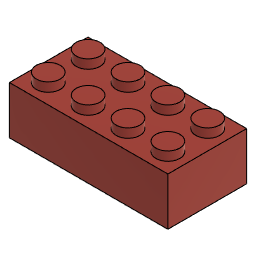
Red Brick v1 (Autodesk Fusion 360 design; units mm, degrees)
Autodesk Fusion 360 part; units mm, degrees
sketch "side" plane through (0, 0, 0) normal (1, 0, 0) x (0, 1, 0)
  line L0 (0, 0) -> (15.8, 0)
  line L1 (15.8, 0) -> (15.8, 9.6)
  line L2 (15.8, 9.6) -> (0, 9.6)
  line L3 (0, 9.6) -> (0, 0)
  dimension "d1" = 15.8
  dimension "d2" = 9.6
  constraint horizontal L0
  constraint vertical L1
  constraint horizontal L2
  constraint vertical L3
  constraint coincident L0.start L3.end
  measures "d1" distance of L0.start L0.end
  measures "d2" distance of L0 L2
sketch "top" plane through (0, 0, 0) normal (0, 0, 1) x (1, 0, 0)
  line L0 (0, 0) -> (-31.8, 0)
  line L1 (-31.8, 0) -> (-31.8, 15.8)
  line L2 (-31.8, 15.8) -> (0, 15.8)
  line L3 (0, 15.8) -> (0, 0)
  circle A0 centre (-3.9, 11.9) radius 2.4
  line L4 (0, 15.8) -> (0, 0)
  circle A1 centre (-11.9, 11.9) radius 2.4
  circle A2 centre (-19.9, 11.9) radius 2.4
  circle A3 centre (-27.9, 11.9) radius 2.4
  circle A4 centre (-3.9, 3.9) radius 2.4
  circle A5 centre (-11.9, 3.9) radius 2.4
  circle A6 centre (-19.9, 3.9) radius 2.4
  circle A7 centre (-27.9, 3.9) radius 2.4
  circle A8 centre (-7.9, 7.9) radius 3.255
  circle A9 centre (-7.9, 7.9) radius 2.4
  circle A10 centre (-3.9, 11.9) radius 1.3
  circle A11 centre (-3.9, 3.9) radius 1.3
  circle A12 centre (-11.9, 11.9) radius 1.3
  circle A13 centre (-11.9, 3.9) radius 1.3
  circle A14 centre (-19.9, 11.9) radius 1.3
  circle A15 centre (-19.9, 3.9) radius 1.3
  circle A16 centre (-27.9, 11.9) radius 1.3
  circle A17 centre (-27.9, 3.9) radius 1.3
  circle A18 centre (-15.9, 7.9) radius 3.255
  circle A19 centre (-23.9, 7.9) radius 3.255
  circle A20 centre (-15.9, 7.9) radius 2.4
  circle A21 centre (-23.9, 7.9) radius 2.4
  line L5 (-30.6, 14.6) -> (-1.2, 14.6)
  line L6 (-1.2, 14.6) -> (-1.2, 1.2)
  line L7 (-1.2, 1.2) -> (-30.6, 1.2)
  line L8 (-30.6, 1.2) -> (-30.6, 14.6)
  line L9 (-15.9, 7.9) -> (-15.9, 14.6) construction
  line L10 (-15.9, 7.9) -> (-15.9, 1.2) construction
  line L11 (-16.3, 11.1303) -> (-16.3, 14.6)
  line L12 (-15.5, 11.1303) -> (-15.5, 14.6)
  line L13 (-15.5, 4.6697) -> (-15.5, 1.2)
  line L14 (-16.3, 4.6697) -> (-16.3, 1.2)
  line L15 (-28.2, 14.6) -> (-27.6, 14.6)
  line L16 (-27.6, 14.6) -> (-27.6, 14.4)
  line L17 (-27.6, 14.4) -> (-28.2, 14.4)
  line L18 (-28.2, 14.4) -> (-28.2, 14.6)
  line L19 (-20.2, 14.6) -> (-19.6, 14.6)
  line L20 (-19.6, 14.6) -> (-19.6, 14.4)
  line L21 (-19.6, 14.4) -> (-20.2, 14.4)
  line L22 (-20.2, 14.4) -> (-20.2, 14.6)
  line L23 (-12.2, 14.6) -> (-11.6, 14.6)
  line L24 (-11.6, 14.6) -> (-11.6, 14.4)
  line L25 (-11.6, 14.4) -> (-12.2, 14.4)
  line L26 (-12.2, 14.4) -> (-12.2, 14.6)
  line L27 (-4.2, 14.4) -> (-3.6, 14.4)
  line L28 (-3.6, 14.4) -> (-3.6, 14.6)
  line L29 (-3.6, 14.6) -> (-4.2, 14.6)
  line L30 (-4.2, 14.6) -> (-4.2, 14.4)
  line L31 (-1.4, 12.2) -> (-1.2, 12.2)
  line L32 (-1.2, 12.2) -> (-1.2, 11.6)
  line L33 (-1.2, 11.6) -> (-1.4, 11.6)
  line L34 (-1.4, 11.6) -> (-1.4, 12.2)
  line L35 (-1.4, 4.2) -> (-1.2, 4.2)
  line L36 (-1.2, 4.2) -> (-1.2, 3.6)
  line L37 (-1.2, 3.6) -> (-1.4, 3.6)
  line L38 (-1.4, 3.6) -> (-1.4, 4.2)
  line L39 (-4.2, 1.4) -> (-3.6, 1.4)
  line L40 (-3.6, 1.4) -> (-3.6, 1.2)
  line L41 (-3.6, 1.2) -> (-4.2, 1.2)
  line L42 (-4.2, 1.2) -> (-4.2, 1.4)
  line L43 (-11.6, 1.4) -> (-12.2, 1.4)
  line L44 (-12.2, 1.4) -> (-12.2, 1.2)
  line L45 (-12.2, 1.2) -> (-11.6, 1.2)
  line L46 (-11.6, 1.2) -> (-11.6, 1.4)
  line L47 (-19.6, 1.4) -> (-20.2, 1.4)
  line L48 (-20.2, 1.4) -> (-20.2, 1.2)
  line L49 (-20.2, 1.2) -> (-19.6, 1.2)
  line L50 (-19.6, 1.2) -> (-19.6, 1.4)
  line L51 (-27.6, 1.4) -> (-28.2, 1.4)
  line L52 (-28.2, 1.4) -> (-28.2, 1.2)
  line L53 (-28.2, 1.2) -> (-27.6, 1.2)
  line L54 (-27.6, 1.2) -> (-27.6, 1.4)
  line L55 (-30.4, 4.2) -> (-30.6, 4.2)
  line L56 (-30.6, 4.2) -> (-30.6, 3.6)
  line L57 (-30.6, 3.6) -> (-30.4, 3.6)
  line L58 (-30.4, 3.6) -> (-30.4, 4.2)
  line L59 (-30.4, 12.2) -> (-30.6, 12.2)
  line L60 (-30.6, 12.2) -> (-30.6, 11.6)
  line L61 (-30.6, 11.6) -> (-30.4, 11.6)
  line L62 (-30.4, 11.6) -> (-30.4, 12.2)
  dimension "d3" = 31.8
  dimension "d4" = 15.8
  dimension "d5" = 4.8
  dimension "d6" = 3.9
  dimension "d7" = 3.9
  dimension "d8" = 4.8
  dimension "d9" = 4.8
  dimension "d10" = 4.8
  dimension "d11" = 4.8
  dimension "d12" = 4.8
  dimension "d13" = 4.8
  dimension "d14" = 4.8
  dimension "d15" = 3.9
  dimension "d16" = 3.9
  dimension "d17" = 3.9
  dimension "d18" = 8
  dimension "d19" = 8
  dimension "d20" = 8
  dimension "d21" = 8
  dimension "d22" = 8
  dimension "d23" = 8
  dimension "d24" = 3.9
  dimension "d25" = 8
  dimension "d26" = 8
  dimension "d27" = 8
  dimension "d28" = 8
  dimension "d29" = 6.51
  dimension "d30" = 7.9
  dimension "d31" = 7.9
  dimension "d32" = 4.8
  dimension "d33" = 2.6
  dimension "d34" = 2.6
  dimension "d35" = 2.6
  dimension "d36" = 2.6
  dimension "d37" = 2.6
  dimension "d38" = 2.6
  dimension "d39" = 2.6
  dimension "d40" = 2.6
  dimension "d41" = 6.51
  dimension "d42" = 6.51
  dimension "d43" = 8
  dimension "d44" = 7.9
  dimension "d45" = 8
  dimension "d46" = 7.9
  dimension "d47" = 4.8
  dimension "d48" = 4.8
  dimension "d49" = 1.2
  dimension "d50" = 1.2
  dimension "d51" = 1.2
  dimension "d52" = 1.2
  dimension "d53" = 0.8
  dimension "d54" = 0.4
  dimension "d55" = 0.4
  dimension "d56" = 0.8
  dimension "d57" = 0.6
  dimension "d58" = 0.2
  dimension "d60" = 0.6
  dimension "d61" = 0.3
  dimension "d62" = 0.6
  dimension "d63" = 0.3
  dimension "d64" = 0.6
  dimension "d65" = 0.3
  dimension "d66" = 0.6
  dimension "d67" = 0.3
  dimension "d68" = 0.6
  dimension "d69" = 0.6
  dimension "d70" = 0.6
  dimension "d71" = 0.6
  dimension "d72" = 0.6
  dimension "d73" = 0.6
  dimension "d74" = 0.3
  dimension "d75" = 0.6
  constraint horizontal L0
  constraint vertical L1
  constraint horizontal L2
  constraint vertical L3
  constraint coincident L0.start L3.end
  constraint concentric A8 A9
  constraint concentric A0 A10
  constraint concentric A4 A11
  constraint concentric A1 A12
  constraint concentric A5 A13
  constraint concentric A2 A14
  constraint concentric A6 A15
  constraint concentric A3 A16
  constraint concentric A7 A17
  constraint concentric A18 A20
  constraint concentric A19 A21
  constraint horizontal L5
  constraint vertical L6
  constraint horizontal L7
  constraint vertical L8
  constraint coincident A18.centre A20.centre
  constraint midpoint L5 L9.end
  constraint midpoint L7 L10.end
  constraint coincident A18 L11.start
  constraint coincident L5 L11.end
  constraint perpendicular L5 L11
  constraint coincident A18 L12.start
  constraint coincident L5 L12.end
  constraint perpendicular L5 L12
  constraint coincident A18 L13.start
  constraint coincident L7 L13.end
  constraint perpendicular L7 L13
  constraint coincident A18 L14.start
  constraint coincident L7 L14.end
  constraint perpendicular L7 L14
  constraint horizontal L15
  constraint vertical L16
  constraint horizontal L17
  constraint vertical L18
  constraint coincident L5 L15.start
  constraint horizontal L19
  constraint vertical L20
  constraint horizontal L21
  constraint vertical L22
  constraint coincident L5 L19.start
  constraint horizontal L23
  constraint vertical L24
  constraint horizontal L25
  constraint vertical L26
  constraint coincident L5 L23.start
  constraint horizontal L27
  constraint vertical L28
  constraint horizontal L29
  constraint vertical L30
  constraint horizontal L31
  constraint vertical L32
  constraint horizontal L33
  constraint vertical L34
  constraint horizontal L35
  constraint vertical L36
  constraint horizontal L37
  constraint vertical L38
  constraint horizontal L39
  constraint vertical L40
  constraint horizontal L41
  constraint vertical L42
  constraint horizontal L43
  constraint vertical L44
  constraint horizontal L45
  constraint vertical L46
  constraint horizontal L47
  constraint vertical L48
  constraint horizontal L49
  constraint vertical L50
  constraint coincident L7 L48.end
  constraint horizontal L51
  constraint vertical L52
  constraint horizontal L53
  constraint vertical L54
  constraint horizontal L55
  constraint vertical L56
  constraint horizontal L57
  constraint vertical L58
  constraint horizontal L59
  constraint vertical L60
  constraint horizontal L61
  constraint vertical L62
  measures "d3" distance of L0.start L0.end
  measures "d4" distance of L0.start L2.end
  measures "d5" diameter of A0
  measures "d6" distance of L2 A0.centre
  measures "d7" distance of A0.centre L4
  measures "d8" diameter of A1
  measures "d9" diameter of A2
  measures "d10" diameter of A3
  measures "d11" diameter of A4
  measures "d12" diameter of A5
  measures "d13" diameter of A6
  measures "d14" diameter of A7
  measures "d15" distance of L2 A1.centre
  measures "d16" distance of L2 A2.centre
  measures "d17" distance of L2 A3.centre
  measures "d18" horizontal distance of A4.centre A5.centre
  measures "d19" horizontal distance of A1.centre A4.centre
  measures "d20" distance of A1.centre A2.centre
  measures "d21" distance of A2.centre A3.centre
  measures "d22" horizontal distance of A6.centre A7.centre
  measures "d23" horizontal distance of A5.centre A6.centre
  measures "d24" distance of L4 A4.centre
  measures "d25" distance of A3.centre A7.centre
  measures "d26" distance of A0.centre A4.centre
  measures "d27" distance of A1.centre A5.centre
  measures "d28" distance of A2.centre A6.centre
  measures "d29" diameter of A8
  measures "d30" distance of L2 A8.centre
  measures "d31" distance of L4 A8.centre
  measures "d32" diameter of A9
  measures "d33" diameter of A10
  measures "d34" diameter of A11
  measures "d35" diameter of A12
  measures "d36" diameter of A13
  measures "d37" diameter of A14
  measures "d38" diameter of A15
  measures "d39" diameter of A16
  measures "d40" diameter of A17
  measures "d41" diameter of A18
  measures "d42" diameter of A19
  measures "d43" horizontal distance of A8.centre A18.centre
  measures "d44" distance of L2 A18.centre
  measures "d45" horizontal distance of A18.centre A19.centre
  measures "d46" distance of L2 A19.centre
  measures "d47" diameter of A20
  measures "d48" diameter of A21
  measures "d49" distance of L1 L8
  measures "d50" distance of L4 L6
  measures "d51" distance of L2 L5
  measures "d52" distance of L0 L7
  measures "d53" distance of L11 L12
  measures "d54" distance of L9 L12
  measures "d55" distance of L10 L13
  measures "d56" distance of L13 L14
  measures "d57" distance of L15.start L15.end
  measures "d58" distance of L15 L17
  measures "d60" distance of L19.start L19.end
  measures "d61" distance of A2.centre L20
  measures "d62" distance of L23.start L23.end
  measures "d63" distance of A1.centre L24
  measures "d64" distance of L27.start L27.end
  measures "d65" distance of A0.centre L28
  measures "d66" distance of L31.start L33.end
  measures "d67" distance of A0.centre L31
  measures "d68" distance of L35.start L37.end
  measures "d69" distance of L39.start L39.end
  measures "d70" distance of L43.start L43.end
  measures "d71" distance of L47.start L47.end
  measures "d72" distance of L51.start L51.end
  measures "d73" distance of L55.start L57.end
  measures "d74" distance of A7.centre L55
  measures "d75" distance of L59.start L61.end
extrude "Extrude1" add sketch "top" along normal blind 9.6 contours L0 L1 L2 L3 L4 | L5 L23 L24 L25 L26 | L5 L19 L20 L21 L22 | L7 L43 L44 L45 L46 | L5 L27 L28 L29 L30 | L7 L47 L48 L49 L50 | L5 L15 L16 L17 L18 | L7 L39 L40 L41 L42 | L7 L51 L52 L53 L54 | L6 L31 L32 L33 L34 | L8 L59 L60 L61 L62 | L6 L35 L36 L37 L38 | L8 L55 L56 L57 L58 makes body 1
extrude "Extrude2" add sketch "top" along normal blind 9.6 and the other way blind -8.6 contours A0 | A4 | A1 A5 A8 A18 L5 L6 L7 L12 L13 L24 L25 L26 L27 L28 L30 L31 L33 L34 L35 L37 L38 L39 L40 L42 L43 L44 L46 | A8 | A1 A5 A8 A18 | A1 | A18 | A5 | A18 L5 L11 L12 | A7 | A3 | A2 A6 A18 A19 L5 L7 L8 L11 L14 L16 L17 L18 L20 L21 L22 L47 L48 L50 L51 L52 L54 L55 L57 L58 L59 L61 L62 | A18 L7 L13 L14 | A2 A6 A18 A19 | A2 | A19 | A6 | A9 | A20 | A21 bodies 1
extrude "Extrude3" add sketch "top" along normal blind 9.6 and the other way blind -11.4 contours A0 | A4 | A1 | A5 | A7 | A3 | A2 | A6 | A10 | A11 | A12 | A13 | A14 | A15 | A16 | A17 bodies 1
extrude "Extrude4" cut sketch "top" along normal blind 10.3 and the other way blind -9.6 contours A10 | A11 | A12 | A13 | A14 | A15 | A16 | A17 bodies 1
extrude "Extrude5" add sketch "top" along normal blind 8.6 contours A8 | A18 | A19 bodies 1
extrude "Extrude6" add sketch "top" along normal blind 8.6 and the other way blind -2.3 contours A18 L5 L11 L12 | A18 L7 L13 L14 bodies 1
copy_body "Body->Comp1" bodies 1 removing the originals makes body 2 in component "Piesa Lego 4x2"
component "Piesa Lego 4x2" placed x (1, 0, 0) y (0, 1, 0) z (0, 0, 1) at (0, 0, 0)
equation "d84 = -9.6 mm - 1.8 mm"
equation "d86 = 8.60 mm + 1.7 mm"
named bodies: "Piesa Lego 4x2"
